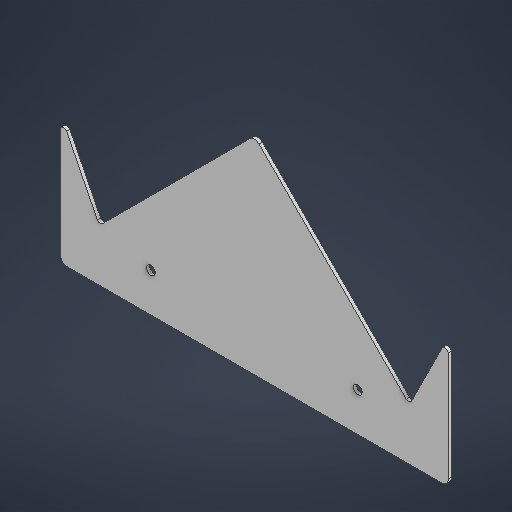
# Autodesk Inventor part: longgoalaligner
Saved by Autodesk Inventor 2026.1 (Build 301233000, 233)
## iProperties
Created: 2026-03-05
Part Number: longgoalaligner
Material: Generic
Document SubType Name: Modeling
Designer: roejo
Density: 1 g/cm^3
Appearance: Default
Author: roejo
Autodesk Inventor part; units mm, degrees
ref_plane "YZ Plane" through (0, 0, 0) normal (1, 0, 0) x (0, 1, 0)
ref_plane "XZ Plane" through (0, 0, 0) normal (0, 1, 0) x (-1, 0, 0)
ref_plane "XY Plane" through (0, 0, 0) normal (0, 0, 1) x (1, 0, 0)
sketch "Sketch1" plane through (0, 0, 0) normal (0, 0, 1) x (1, 0, 0)
  line L0 (0, 0) -> (0, 76.2)
  line L1 (-2.2451, 73.9549) -> (-74.6426, 1.5574)
  line L2 (2.2451, 73.9549) -> (74.6426, 1.5574)
  line L3 (0, 0) -> (95.25, 0)
  line L4 (0, 0) -> (-95.25, 0)
  line L5 (95.25, 0) -> (95.25, 31.3752)
  line L6 (92.2426, 32.0852) -> (77.185, 1.97)
  line L7 (-95.25, 0) -> (-95.25, 31.3752)
  line L8 (-92.2426, 32.0852) -> (-77.185, 1.97)
  line L9 (-95.25, 0) -> (-95.25, -22.225)
  line L10 (-92.075, -25.4) -> (92.075, -25.4)
  line L11 (95.25, -22.225) -> (95.25, 0)
  arc A0 (2.2451, 73.9549) -> (-2.2451, 73.9549) centre (0, 71.7099) ccw
  arc A1 (92.075, -25.4) -> (95.25, -22.225) centre (92.075, -22.225) ccw
  arc A2 (-95.25, -22.225) -> (-92.075, -25.4) centre (-92.075, -22.225) ccw
  arc A3 (-77.185, 1.97) -> (-74.6426, 1.5574) centre (-75.7651, 2.68) ccw
  arc A4 (-92.2426, 32.0852) -> (-95.25, 31.3752) centre (-93.6625, 31.3752) ccw
  arc A5 (95.25, 31.3752) -> (92.2426, 32.0852) centre (93.6625, 31.3752) ccw
  arc A6 (74.6426, 1.5574) -> (77.185, 1.97) centre (75.7651, 2.68) ccw
  circle A7 centre (50.8, -6.35) radius 2.1844
  circle A8 centre (-50.8, -6.35) radius 2.1844
  point P0 (-76.2, 0)
  point P1 (76.2, 0)
  point P2 (95.25, 38.1)
  point P3 (-95.25, 38.1)
  point P4 (-95.25, -25.4)
  dimension "d0" = 76.2
  dimension "d3" = 45
  dimension "d4" = 45
  dimension "d5" = 95.25
  dimension "d6" = 95.25
  dimension "d7" = 38.1
  dimension "d8" = 38.1
  dimension "d9" = 25.4
  dimension "d10" = 3.175
  dimension "d11" = 3.175
  dimension "d12" = 1.5875
  dimension "d13" = 4.3688
  dimension "d14" = 50.8
  dimension "d15" = 6.35
  dimension "d16" = 4.3688
  dimension "d17" = 50.8
  dimension "d18" = 6.35
  constraints: 24 end point, 14 point on circle, 14 point on line, 14 tangent, 9 centre point, 4 equal radius, 3 perpendicular, 3 vertical, 2 horizontal
  measures "d0" distance of L0.start L0.end
  measures "d3" angle of L0 L2
  measures "d4" angle of L0 L1
  measures "d5" distance of L0.start L3.end
  measures "d6" distance of L0.start L4.end
  measures "d7" distance of L3.end point (95.25, 38.1)
  measures "d8" distance of L4.end point (-95.25, 38.1)
  measures "d9" distance of L4.end point (-95.25, -25.4)
  measures "d10" radius of A0
  measures "d11" radius of A1
  measures "d12" radius of A3
  measures "d13" diameter of A7
  measures "d14" horizontal distance of L0.start A7.centre
  measures "d15" distance from line of L3 A7.centre
  measures "d16" diameter of A8
  measures "d17" horizontal distance of L0.start A8.centre
  measures "d18" distance from line of L4 A8.centre
extrude "Extrusion1" add sketch "Sketch1" along normal blind 1.5875
body "Solid1"
